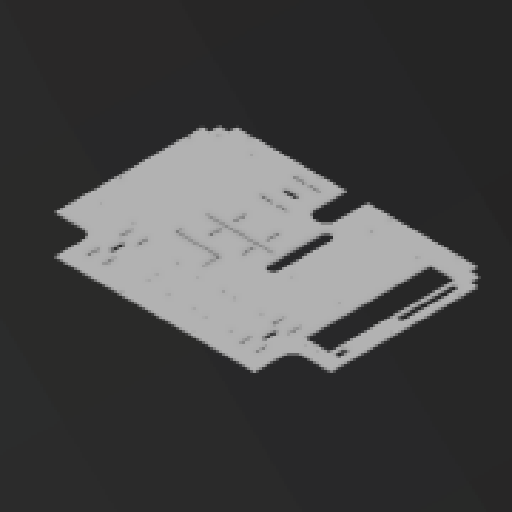
# Autodesk Inventor part: BasePlate
Saved by Autodesk Inventor 2023.2 (Build 272271000, 271)
## iProperties
Created: 2020-05-08
Part Number: BasePlate
Material: Aluminum 6061
Document SubType Name: Modeling
Designer: Remo
Mass: 4435.74 g
Surface Area: 3861.35 cm^2
Volume: 565.063 cm^3
Density: 2.7 g/cm^3
Appearance: Aluminum - Dark
Description: LaserTeileOnline / 3mm Aluminum / Base Plate
Author: Remo
Revision Number: 1
Autodesk Inventor part; units mm, degrees
ref_plane "YZ Plane" through (0, 0, 0) normal (1, 0, 0) x (0, 1, 0)
ref_plane "XZ Plane" through (0, 0, 0) normal (0, 1, 0) x (-1, 0, 0)
ref_plane "XY Plane" through (0, 0, 0) normal (0, 0, 1) x (1, 0, 0)
sketch "Sketch1" plane through (0, 0, 0) normal (0, 0, 1) x (1, 0, 0)
  line L0 (-412.8165, 301.8597) -> (87.1835, 301.8597) projected
  line L1 (-427.8165, 301.8597) -> (-412.8165, 301.8597) projected
  line L2 (-427.8165, 286.8597) -> (-427.8165, 301.8597) projected
  line L3 (-427.8165, -73.1403) -> (-427.8165, 286.8597) projected
  line L4 (-412.8165, 286.8597) -> (-427.8165, 286.8597) projected
  line L5 (-412.8165, 286.8597) -> (-427.8165, 286.8597) projected
  line L6 (-412.8165, 301.8597) -> (-412.8165, 286.8597) projected
  line L7 (-427.8165, 301.8597) -> (-412.8165, 301.8597) projected
  line L8 (-427.8165, 286.8597) -> (-427.8165, 301.8597) projected
  line L9 (-412.8165, -88.1403) -> (-412.8165, -73.1403) projected
  line L10 (-412.8165, -73.1403) -> (-427.8165, -73.1403) projected
  line L11 (-427.8165, -88.1403) -> (-427.8165, -73.1403) projected
  line L12 (-412.8165, -88.1403) -> (-427.8165, -88.1403) projected
  line L13 (-412.8165, -73.1403) -> (-412.8165, 286.8597) projected
  line L14 (87.1835, -73.1403) -> (-412.8165, -73.1403) projected
  line L15 (87.1835, -88.1403) -> (-412.8165, -88.1403) projected
  line L16 (102.1835, -88.1403) -> (102.1835, -73.1403) projected
  line L17 (102.1835, -73.1403) -> (87.1835, -73.1403) projected
  line L18 (87.1835, -88.1403) -> (87.1835, -73.1403) projected
  line L19 (102.1835, -88.1403) -> (87.1835, -88.1403) projected
  line L20 (87.1835, -73.1403) -> (87.1835, 286.8597) projected
  line L21 (102.1835, -73.1403) -> (102.1835, 286.8597) projected
  line L22 (87.1835, 286.8597) -> (102.1835, 286.8597) projected
  line L23 (102.1835, 286.8597) -> (102.1835, 301.8597) projected
  line L24 (87.1835, 301.8597) -> (102.1835, 301.8597) projected
  line L25 (87.1835, 286.8597) -> (87.1835, 301.8597) projected
  line L26 (87.1835, 286.8597) -> (-412.8165, 286.8597) projected
  line L27 (-312.8165, -73.1403) -> (-312.8165, 286.8597) projected
  line L28 (-297.8165, -73.1403) -> (-297.8165, 286.8597) projected
  line L29 (-12.8165, -73.1403) -> (-12.8165, 286.8597) projected
  line L30 (-27.8165, -73.1403) -> (-27.8165, 286.8597) projected
  line L31 (-425.8165, -71.1403) -> (-410.8165, -71.1403)
  line L32 (-410.8165, -71.1403) -> (-410.8165, -86.1403)
  line L33 (-410.8165, -86.1403) -> (85.1835, -86.1403)
  line L34 (85.1835, -86.1403) -> (85.1835, -71.1403)
  line L35 (85.1835, -71.1403) -> (100.1835, -71.1403)
  line L36 (100.1835, -71.1403) -> (100.1835, 284.8597)
  line L37 (100.1835, 284.8597) -> (85.1835, 284.8597)
  line L38 (85.1835, 284.8597) -> (85.1835, 299.8597)
  line L39 (85.1835, 299.8597) -> (-410.8165, 299.8597)
  line L40 (-410.8165, 299.8597) -> (-410.8165, 284.8597)
  line L41 (-410.8165, 284.8597) -> (-425.8165, 284.8597)
  line L42 (-425.8165, 284.8597) -> (-425.8165, -71.1403)
  point P0 (0, 0)
  dimension "d2" = 2
  dimension "d3" = 2
  dimension "d4" = 2
  dimension "d5" = 2
  dimension "d6" = 2
  dimension "d7" = 2
  dimension "d8" = 2
  dimension "d9" = 2
  dimension "d10" = 2
  dimension "d11" = 2
  dimension "d12" = 2
  dimension "d13" = 2
  constraints: 24 end point, 7 perpendicular, 4 parallel, 1 horizontal
  measures "d2" distance between parallel lines of L10 L31
  measures "d3" distance between parallel lines of L3 L42
  measures "d4" distance between parallel lines of L9 L32
  measures "d5" distance between parallel lines of L15 L33
  measures "d6" distance between parallel lines of L34 L18
  measures "d7" distance between parallel lines of L17 L35
  measures "d8" distance between parallel lines of L21 L36
  measures "d9" distance between parallel lines of L22 L37
  measures "d10" distance between parallel lines of L25 L38
  measures "d11" distance between parallel lines of L0 L39
  measures "d12" distance between parallel lines of L6 L40
  measures "d13" distance between parallel lines of L4 L41
extrude "Extrusion1" add sketch "Sketch1" along normal blind 3 contours L41 L40 L26 L27 L14 L32 L31 L13 | L13 L31 L42 L41 | L40 L39 L38 L26 | L37 L36 L35 L20 | L20 L35 L34 L14 L29 L26 L38 L37 | L26 L28 L14 L27 | L29 L14 L30 L26 | L26 L30 L14 L28 | L14 L34 L33 L32
sketch "Sketch3" plane through (0, 0, 3) normal (0, 0, 1) x (1, 0, 0)
  line L0 (100.1835, -71.1403) -> (100.1835, 284.8597) projected
  line L1 (-425.8165, 284.8597) -> (-425.8165, -71.1403) projected
  line L2 (-425.8165, -71.1403) -> (-410.8165, -71.1403) projected
  line L3 (-410.8165, 284.8597) -> (-425.8165, 284.8597) projected
  line L4 (85.1835, -86.1403) -> (85.1835, -71.1403) projected
  line L5 (-410.8165, 299.8597) -> (-410.8165, 284.8597) projected
  line L6 (-410.8165, -86.1403) -> (85.1835, -86.1403) projected
  line L7 (85.1835, 299.8597) -> (-410.8165, 299.8597) projected
  point P0 (0, 0)
  point P1 (94.6835, -21.1403)
  point P2 (94.6835, 106.8597)
  point P3 (94.6835, 234.8597)
  point P4 (-420.3165, 234.8597)
  point P5 (-420.3165, 106.8597)
  point P6 (-420.3165, -21.1403)
  point P7 (35.1835, -80.6403)
  point P8 (-94.8165, -80.6403)
  point P9 (-230.8165, -80.6403)
  point P10 (-360.8165, -80.6403)
  point P11 (-360.8165, 294.3597)
  point P12 (-230.8165, 294.3597)
  point P13 (-94.8165, 294.3597)
  point P14 (35.1835, 294.3597)
  dimension "d18" = 5.5
  dimension "d19" = 5.5
  dimension "d20" = 50
  dimension "d21" = 50
  dimension "d22" = 356
  dimension "d23" = 178
  dimension "d24" = 50
  dimension "d25" = 50
  dimension "d26" = 5.5
  dimension "d27" = 5.5
  dimension "d28" = 180
  dimension "d29" = 180
  constraints: 9 horizontal alignment, 8 vertical alignment
  measures "d18" distance from line of L0 point (94.684, -21.14)
  measures "d19" distance from line of L1 point (-420.316, -21.14)
  measures "d20" distance from line of L2 point (-420.316, -21.14)
  measures "d21" distance from line of L3 point (-420.316, 234.86)
  measures "d22" distance of L1.start L1.end
  measures "d23" distance from line of L2 point (-420.316, 106.86)
  measures "d24" distance from line of L4 point (35.184, -80.64)
  measures "d25" distance from line of L5 point (-360.816, 294.36)
  measures "d26" distance from line of L6 point (35.184, -80.64)
  measures "d27" distance from line of L7 point (35.184, 294.36)
  measures "d28" horizontal distance of L6.start point (-230.816, -80.64)
  measures "d29" distance from line of L4 point (-94.816, -80.64)
hole "FrameMountHoles" at (94.6835, -21.1403, 3) at (94.6835, 106.8597, 3) at (94.6835, 234.8597, 3) at (-420.3165, 234.8597, 3) at (-420.3165, 106.8597, 3) at (-420.3165, -21.1403, 3) at (35.1835, -80.6403, 3) at (-94.8165, -80.6403, 3) at (-230.8165, -80.6403, 3) at (-360.8165, -80.6403, 3) at (-360.8165, 294.3597, 3) at (-230.8165, 294.3597, 3) at (-94.8165, 294.3597, 3) at (35.1835, 294.3597, 3) direction (0, 0, -1) diameter 4 depth 8 tip angle 118
sketch "Sketch10" plane through (0, 0, 3) normal (0, 0, 1) x (1, 0, 0)
  circle A0 centre (-94.8165, 294.3597) radius 2 projected
  circle A1 centre (-360.8165, 294.3597) radius 2 projected
  circle A2 centre (-230.8165, -80.6403) radius 2 projected
  circle A3 centre (35.1835, -80.6403) radius 2 projected
  circle A4 centre (-420.3165, 106.8597) radius 2 projected
  circle A5 centre (94.6835, 234.8597) radius 2 projected
  circle A6 centre (94.6835, -21.1403) radius 2 projected
  circle A7 centre (94.6835, 106.8597) radius 2 projected
  circle A8 centre (-420.3165, 234.8597) radius 2 projected
  circle A9 centre (-420.3165, -21.1403) radius 2 projected
  circle A10 centre (-94.8165, -80.6403) radius 2 projected
  circle A11 centre (-360.8165, -80.6403) radius 2 projected
  circle A12 centre (-230.8165, 294.3597) radius 2 projected
  circle A13 centre (35.1835, 294.3597) radius 2 projected
  line L0 (-425.8165, -71.1403) -> (-410.8165, -71.1403) projected
  line L1 (-410.8165, -71.1403) -> (-410.8165, -86.1403) projected
  line L2 (-410.8165, -86.1403) -> (85.1835, -86.1403) projected
  line L3 (85.1835, -86.1403) -> (85.1835, -71.1403) projected
  line L4 (85.1835, -71.1403) -> (100.1835, -71.1403) projected
  line L5 (100.1835, -71.1403) -> (100.1835, 284.8597) projected
  line L6 (100.1835, 284.8597) -> (85.1835, 284.8597) projected
  line L7 (85.1835, 284.8597) -> (85.1835, 299.8597) projected
  line L8 (85.1835, 299.8597) -> (-410.8165, 299.8597) projected
  line L9 (-410.8165, 299.8597) -> (-410.8165, 284.8597) projected
  line L10 (-410.8165, 284.8597) -> (-425.8165, 284.8597) projected
  line L11 (-425.8165, 284.8597) -> (-425.8165, -71.1403) projected
  line L12 (100.1835, -71.1403) -> (100.1835, 284.8597) projected
  line L13 (85.1835, 284.8597) -> (100.1835, 284.8597)
  line L14 (100.1835, 284.8597) -> (100.1835, 266.8597)
  line L15 (100.1835, 266.8597) -> (85.1835, 266.8597)
  line L16 (85.1835, 266.8597) -> (85.1835, 284.8597)
  line L17 (85.1835, 284.8597) -> (67.1835, 284.8597)
  line L18 (67.1835, 284.8597) -> (67.1835, 299.8597)
  line L19 (67.1835, 299.8597) -> (85.1835, 299.8597)
  line L20 (85.1835, 299.8597) -> (85.1835, 284.8597)
  line L21 (-410.8165, 284.8597) -> (-392.8165, 284.8597)
  line L22 (-392.8165, 284.8597) -> (-392.8165, 299.8597)
  line L23 (-392.8165, 299.8597) -> (-410.8165, 299.8597)
  line L24 (-410.8165, 299.8597) -> (-410.8165, 284.8597)
  line L25 (-410.8165, 284.8597) -> (-425.8165, 284.8597)
  line L26 (-425.8165, 284.8597) -> (-425.8165, 266.8597)
  line L27 (-425.8165, 266.8597) -> (-410.8165, 266.8597)
  line L28 (-410.8165, 266.8597) -> (-410.8165, 284.8597)
  line L29 (-410.8165, -71.1403) -> (-425.8165, -71.1403)
  line L30 (-425.8165, -71.1403) -> (-425.8165, -53.1403)
  line L31 (-425.8165, -53.1403) -> (-410.8165, -53.1403)
  line L32 (-410.8165, -53.1403) -> (-410.8165, -71.1403)
  line L33 (-410.8165, -71.1403) -> (-392.8165, -71.1403)
  line L34 (-392.8165, -71.1403) -> (-392.8165, -86.1403)
  line L35 (-392.8165, -86.1403) -> (-410.8165, -86.1403)
  line L36 (-410.8165, -86.1403) -> (-410.8165, -71.1403)
  line L37 (-410.8165, -86.1403) -> (85.1835, -86.1403) projected
  line L38 (85.1835, -71.1403) -> (67.1835, -71.1403)
  line L39 (67.1835, -71.1403) -> (67.1835, -86.1403)
  line L40 (67.1835, -86.1403) -> (85.1835, -86.1403)
  line L41 (85.1835, -86.1403) -> (85.1835, -71.1403)
  line L42 (85.1835, -71.1403) -> (100.1835, -71.1403)
  line L43 (100.1835, -71.1403) -> (100.1835, -53.1403)
  line L44 (100.1835, -53.1403) -> (85.1835, -53.1403)
  line L45 (85.1835, -53.1403) -> (85.1835, -71.1403)
  point P0 (0, 0)
  dimension "d78" = 18
  constraints: 64 end point, 16 parallel, 8 horizontal, 8 perpendicular, 8 point on line, 7 equal length
  measures "d78" distance of L3.end L38.end
extrude "TriCuts" cut sketch "Sketch10" against normal through all contours L11 L31 L32 L0 | L33 L34 L2 L1 | L11 L10 L28 L27 | L39 L38 L3 L2 | L9 L8 L22 L21 | L45 L44 L5 L4 | L8 L7 L17 L18 | L15 L16 L6 L5
sketch "Sketch18" plane through (0, 0, 0) normal (0, 0, -1) x (-1, 0, 0)
  circle A0 centre (-35.1835, 294.3597) radius 2 projected
  circle A1 centre (230.8165, 294.3597) radius 2 projected
  circle A2 centre (360.8165, -80.6403) radius 2 projected
  circle A3 centre (94.8165, -80.6403) radius 2 projected
  circle A4 centre (420.3165, -21.1403) radius 2 projected
  circle A5 centre (420.3165, 234.8597) radius 2 projected
  circle A6 centre (-94.6835, 106.8597) radius 2 projected
  circle A7 centre (-94.6835, -21.1403) radius 2 projected
  circle A8 centre (-94.6835, 234.8597) radius 2 projected
  circle A9 centre (420.3165, 106.8597) radius 2 projected
  circle A10 centre (-35.1835, -80.6403) radius 2 projected
  circle A11 centre (230.8165, -80.6403) radius 2 projected
  circle A12 centre (360.8165, 294.3597) radius 2 projected
  circle A13 centre (94.8165, 294.3597) radius 2 projected
  line L0 (425.8165, 266.8597) -> (410.8165, 266.8597) projected
  line L1 (410.8165, 266.8597) -> (410.8165, 284.8597) projected
  line L2 (410.8165, 284.8597) -> (392.8165, 284.8597) projected
  line L3 (392.8165, 284.8597) -> (392.8165, 299.8597) projected
  line L4 (-67.1835, 299.8597) -> (392.8165, 299.8597) projected
  line L5 (-67.1835, 299.8597) -> (-67.1835, 284.8597) projected
  line L6 (-67.1835, 284.8597) -> (-85.1835, 284.8597) projected
  line L7 (-85.1835, 284.8597) -> (-85.1835, 266.8597) projected
  line L8 (-85.1835, 266.8597) -> (-100.1835, 266.8597) projected
  line L9 (-100.1835, -53.1403) -> (-100.1835, 266.8597) projected
  line L10 (-100.1835, -53.1403) -> (-85.1835, -53.1403) projected
  line L11 (-85.1835, -53.1403) -> (-85.1835, -71.1403) projected
  line L12 (-85.1835, -71.1403) -> (-67.1835, -71.1403) projected
  line L13 (-67.1835, -71.1403) -> (-67.1835, -86.1403) projected
  line L14 (392.8165, -86.1403) -> (-67.1835, -86.1403) projected
  line L15 (392.8165, -86.1403) -> (392.8165, -71.1403) projected
  line L16 (392.8165, -71.1403) -> (410.8165, -71.1403) projected
  line L17 (410.8165, -71.1403) -> (410.8165, -53.1403) projected
  line L18 (410.8165, -53.1403) -> (425.8165, -53.1403) projected
  line L19 (425.8165, 266.8597) -> (425.8165, -53.1403) projected
  circle A14 centre (-47.2571, -33.2139) radius 4 projected
  circle A15 centre (-47.2571, -33.2139) radius 20
  line L20 (-27.2571, -33.2139) -> (-27.2571, -86.1403)
  line L21 (392.8165, -86.1403) -> (-67.1835, -86.1403) projected
  line L22 (-47.2571, -13.2139) -> (-100.1835, -13.2139)
  line L23 (-100.1835, -53.1403) -> (-100.1835, 266.8597) projected
  circle A16 centre (372.89, -33.2139) radius 4 projected
  circle A17 centre (372.89, -33.2139) radius 20
  line L24 (372.89, -13.2139) -> (425.8165, -13.2139)
  line L25 (425.8165, 266.8597) -> (425.8165, -53.1403) projected
  line L26 (352.89, -33.2139) -> (352.89, -86.1403)
  line L27 (392.8165, -86.1403) -> (-67.1835, -86.1403) projected
  circle A18 centre (162.8165, 240.7787) radius 4 projected
  circle A19 centre (162.8165, 240.7787) radius 20
  line L28 (142.8165, 240.7787) -> (142.8165, 299.8597)
  line L29 (-67.1835, 299.8597) -> (392.8165, 299.8597) projected
  line L30 (182.8165, 240.7787) -> (182.8165, 299.8597)
  line L31 (-20.1835, 16.7861) -> (-67.1835, 16.7861)
  line L32 (-67.1835, 16.7861) -> (-67.1835, 256.7861)
  line L33 (-67.1835, 256.7861) -> (-20.1835, 256.7861)
  line L34 (-20.1835, 256.7861) -> (-20.1835, 16.7861)
  line L35 (-75.1835, 16.7861) -> (-85.1835, 16.7861)
  line L36 (-85.1835, 16.7861) -> (-85.1835, 36.7861)
  line L37 (-85.1835, 36.7861) -> (-75.1835, 36.7861)
  line L38 (-75.1835, 36.7861) -> (-75.1835, 16.7861)
  point P0 (0, 0)
  point P1 (352.89, -86.1403)
  dimension "d130" = 40
  dimension "d133" = 33
  dimension "d134" = 47
  dimension "d135" = 30
  dimension "d136" = 240
  dimension "d151" = 15
  dimension "d152" = 10
  dimension "d153" = 20
  constraints: 28 end point, 8 perpendicular, 6 point on circle, 6 point on line, 4 parallel, 4 tangent, 3 centre point, 3 coincident, 2 equal radius, 2 horizontal, 1 horizontal alignment
  measures "d130" diameter of A15
  measures "d133" distance between parallel lines of L23 L32
  measures "d134" distance of L31.start L31.end
  measures "d135" distance between parallel lines of L22 L31
  measures "d136" distance of L31.end L32.end
  measures "d151" distance between parallel lines of L23 L36
  measures "d152" distance of L35.start L35.end
  measures "d153" distance of L37.end L35.start
extrude "Cuts" cut sketch "Sketch18" against normal through all contours L19 L18 L17 L16 L15 L14 L26 A17 L24 | A17 | L30 A19 L28 L4 | L14 L13 L12 L11 L10 L9 L22 A15 L20 | A19 | A15 | A14 | A16 | A18 | L31 L32 L33 L34 | L35 L36 L37 L38
sketch "Sketch19" plane through (0, 0, 0) normal (0, 0, -1) x (-1, 0, 0)
  circle A0 centre (94.8165, 294.3597) radius 2 projected
  circle A1 centre (360.8165, 294.3597) radius 2 projected
  circle A2 centre (230.8165, -80.6403) radius 2 projected
  circle A3 centre (420.3165, 106.8597) radius 2 projected
  circle A4 centre (-94.6835, 234.8597) radius 2 projected
  circle A5 centre (-94.6835, 106.8597) radius 2 projected
  circle A6 centre (420.3165, 234.8597) radius 2 projected
  circle A7 centre (94.8165, -80.6403) radius 2 projected
  circle A8 centre (230.8165, 294.3597) radius 2 projected
  circle A9 centre (-35.1835, 294.3597) radius 2 projected
  line L0 (-67.1835, 16.7861) -> (-67.1835, 256.7861) projected
  line L1 (-67.1835, 256.7861) -> (-20.1835, 256.7861) projected
  line L2 (-20.1835, 256.7861) -> (-20.1835, 16.7861) projected
  line L3 (-20.1835, 16.7861) -> (-67.1835, 16.7861) projected
  line L4 (352.89, -86.1403) -> (352.89, -33.2139) projected
  arc A10 (372.89, -13.2139) -> (352.89, -33.2139) centre (372.89, -33.2139) ccw projected
  line L5 (372.89, -13.2139) -> (425.8165, -13.2139) projected
  line L6 (425.8165, 266.8597) -> (425.8165, -13.2139) projected
  line L7 (425.8165, 266.8597) -> (410.8165, 266.8597) projected
  line L8 (410.8165, 266.8597) -> (410.8165, 284.8597) projected
  line L9 (410.8165, 284.8597) -> (392.8165, 284.8597) projected
  line L10 (392.8165, 284.8597) -> (392.8165, 299.8597) projected
  line L11 (182.8165, 299.8597) -> (392.8165, 299.8597) projected
  line L12 (182.8165, 299.8597) -> (182.8165, 240.7787) projected
  arc A11 (142.8165, 240.7787) -> (182.8165, 240.7787) centre (162.8165, 240.7787) ccw projected
  line L13 (142.8165, 240.7787) -> (142.8165, 299.8597) projected
  line L14 (-67.1835, 299.8597) -> (142.8165, 299.8597) projected
  line L15 (-67.1835, 299.8597) -> (-67.1835, 284.8597) projected
  line L16 (-67.1835, 284.8597) -> (-85.1835, 284.8597) projected
  line L17 (-85.1835, 284.8597) -> (-85.1835, 266.8597) projected
  line L18 (-85.1835, 266.8597) -> (-100.1835, 266.8597) projected
  line L19 (-100.1835, -13.2139) -> (-100.1835, 266.8597) projected
  line L20 (-100.1835, -13.2139) -> (-47.2571, -13.2139) projected
  arc A12 (-27.2571, -33.2139) -> (-47.2571, -13.2139) centre (-47.2571, -33.2139) ccw projected
  line L21 (-27.2571, -33.2139) -> (-27.2571, -86.1403) projected
  line L22 (352.89, -86.1403) -> (-27.2571, -86.1403) projected
  line L23 (-20.1835, 16.7861) -> (-67.1835, 16.7861) projected
  point P0 (0, 0)
  point P1 (-32.6835, 4.7861)
  point P2 (-54.6835, 4.7861)
  point P3 (-43.6835, 12.7861)
  point P4 (-43.6835, 16.7861)
  point P5 (-43.6835, 16.7861)
  dimension "d137" = 12
  dimension "d138" = 4
  dimension "d139" = 22
  dimension "d140" = 11
  constraints: 2 midpoint, 1 horizontal alignment, 1 vertical alignment
  measures "d137" distance from line of L3 point (-32.684, 4.786)
  measures "d138" distance from line of L3 point (-43.684, 12.786)
  measures "d139" distance of point (-54.684, 4.786) point (-32.684, 4.786)
  measures "d140" horizontal distance of point (-43.684, 16.786) point (-54.684, 4.786)
hole "Drag Chain Z" at (32.6835, 4.7861, 0) at (54.6835, 4.7861, 0) at (43.6835, 12.7861, 0) direction (0, 0, 1) diameter 2.8 end through all
sketch "Sketch21" plane through (0, 0, 0) normal (0, 0, -1) x (-1, 0, 0)
  circle A0 centre (32.395, 19.3597) radius 1.75 projected
  circle A1 centre (2.395, 19.3597) radius 1.75 projected
  circle A2 centre (17.395, -12.1403) radius 2.5 projected
  circle A3 centre (32.395, -43.6403) radius 1.75 projected
  circle A4 centre (2.395, -43.6403) radius 1.75 projected
  circle A5 centre (323.2379, -43.6403) radius 1.75 projected
  circle A6 centre (293.2379, -43.6403) radius 1.75 projected
  circle A7 centre (308.2379, -12.1403) radius 2.5 projected
  circle A8 centre (293.2379, 19.3597) radius 1.75 projected
  circle A9 centre (323.2379, 19.3597) radius 1.75 projected
  circle A10 centre (245.8164, 272.3597) radius 1.75 projected
  circle A11 centre (215.8164, 272.3597) radius 1.75 projected
  circle A12 centre (230.8164, 240.8597) radius 2.5 projected
  circle A13 centre (245.8164, 209.3597) radius 1.75 projected
  circle A14 centre (215.8164, 209.3597) radius 1.75 projected
  line L0 (205.8164, 272.3597) -> (225.8164, 272.3597) construction
  line L1 (205.8164, 270.6097) -> (225.8164, 270.6097)
  line L2 (225.8164, 274.1097) -> (205.8164, 274.1097)
  arc A15 (205.8164, 274.1097) -> (205.8164, 270.6097) centre (205.8164, 272.3597) ccw
  arc A16 (225.8164, 270.6097) -> (225.8164, 274.1097) centre (225.8164, 272.3597) ccw
  line L3 (235.8164, 272.3597) -> (255.8164, 272.3597) construction
  line L4 (235.8164, 270.6097) -> (255.8164, 270.6097)
  line L5 (255.8164, 274.1097) -> (235.8164, 274.1097)
  arc A17 (235.8164, 274.1097) -> (235.8164, 270.6097) centre (235.8164, 272.3597) ccw
  arc A18 (255.8164, 270.6097) -> (255.8164, 274.1097) centre (255.8164, 272.3597) ccw
  line L6 (235.8164, 209.3597) -> (255.8164, 209.3597) construction
  line L7 (235.8164, 207.6097) -> (255.8164, 207.6097)
  line L8 (255.8164, 211.1097) -> (235.8164, 211.1097)
  arc A19 (235.8164, 211.1097) -> (235.8164, 207.6097) centre (235.8164, 209.3597) ccw
  arc A20 (255.8164, 207.6097) -> (255.8164, 211.1097) centre (255.8164, 209.3597) ccw
  line L9 (205.8164, 209.3597) -> (225.8164, 209.3597) construction
  line L10 (205.8164, 207.6097) -> (225.8164, 207.6097)
  line L11 (225.8164, 211.1097) -> (205.8164, 211.1097)
  arc A21 (205.8164, 211.1097) -> (205.8164, 207.6097) centre (205.8164, 209.3597) ccw
  arc A22 (225.8164, 207.6097) -> (225.8164, 211.1097) centre (225.8164, 209.3597) ccw
  line L12 (220.8164, 240.8597) -> (240.8164, 240.8597) construction
  line L13 (220.8164, 236.8597) -> (240.8164, 236.8597)
  line L14 (240.8164, 244.8597) -> (220.8164, 244.8597)
  arc A23 (220.8164, 244.8597) -> (220.8164, 236.8597) centre (220.8164, 240.8597) ccw
  arc A24 (240.8164, 236.8597) -> (240.8164, 244.8597) centre (240.8164, 240.8597) ccw
  line L15 (293.2379, 9.3597) -> (293.2379, 29.3597) construction
  line L16 (291.4879, 9.3597) -> (291.4879, 29.3597)
  line L17 (294.9879, 29.3597) -> (294.9879, 9.3597)
  arc A25 (291.4879, 9.3597) -> (294.9879, 9.3597) centre (293.2379, 9.3597) ccw
  arc A26 (294.9879, 29.3597) -> (291.4879, 29.3597) centre (293.2379, 29.3597) ccw
  line L18 (323.2379, 29.3597) -> (323.2379, 9.3597) construction
  line L19 (324.9879, 29.3597) -> (324.9879, 9.3597)
  line L20 (321.4879, 9.3597) -> (321.4879, 29.3597)
  arc A27 (324.9879, 29.3597) -> (321.4879, 29.3597) centre (323.2379, 29.3597) ccw
  arc A28 (321.4879, 9.3597) -> (324.9879, 9.3597) centre (323.2379, 9.3597) ccw
  line L21 (308.2379, -22.1403) -> (308.2379, -2.1403) construction
  line L22 (312.2379, -22.1403) -> (312.2379, -2.1403)
  line L23 (304.2379, -2.1403) -> (304.2379, -22.1403)
  arc A29 (304.2379, -22.1403) -> (312.2379, -22.1403) centre (308.2379, -22.1403) ccw
  arc A30 (312.2379, -2.1403) -> (304.2379, -2.1403) centre (308.2379, -2.1403) ccw
  line L24 (293.2379, -53.6403) -> (293.2379, -33.6403) construction
  line L25 (294.9879, -53.6403) -> (294.9879, -33.6403)
  line L26 (291.4879, -33.6403) -> (291.4879, -53.6403)
  arc A31 (291.4879, -53.6403) -> (294.9879, -53.6403) centre (293.2379, -53.6403) ccw
  arc A32 (294.9879, -33.6403) -> (291.4879, -33.6403) centre (293.2379, -33.6403) ccw
  line L27 (323.2379, -53.6403) -> (323.2379, -33.6403) construction
  line L28 (321.4879, -53.6403) -> (321.4879, -33.6403)
  line L29 (324.9879, -33.6403) -> (324.9879, -53.6403)
  arc A33 (321.4879, -53.6403) -> (324.9879, -53.6403) centre (323.2379, -53.6403) ccw
  arc A34 (324.9879, -33.6403) -> (321.4879, -33.6403) centre (323.2379, -33.6403) ccw
  line L30 (17.395, -22.1403) -> (17.395, -2.1403) construction
  line L31 (13.395, -22.1403) -> (13.395, -2.1403)
  line L32 (21.395, -2.1403) -> (21.395, -22.1403)
  arc A35 (13.395, -22.1403) -> (21.395, -22.1403) centre (17.395, -22.1403) ccw
  arc A36 (21.395, -2.1403) -> (13.395, -2.1403) centre (17.395, -2.1403) ccw
  line L33 (32.395, 9.3597) -> (32.395, 29.3597) construction
  line L34 (30.645, 9.3597) -> (30.645, 29.3597)
  line L35 (34.145, 29.3597) -> (34.145, 9.3597)
  arc A37 (30.645, 9.3597) -> (34.145, 9.3597) centre (32.395, 9.3597) ccw
  arc A38 (34.145, 29.3597) -> (30.645, 29.3597) centre (32.395, 29.3597) ccw
  line L36 (2.395, 9.3597) -> (2.395, 29.3597) construction
  line L37 (0.645, 9.3597) -> (0.645, 29.3597)
  line L38 (4.145, 29.3597) -> (4.145, 9.3597)
  arc A39 (0.645, 9.3597) -> (4.145, 9.3597) centre (2.395, 9.3597) ccw
  arc A40 (4.145, 29.3597) -> (0.645, 29.3597) centre (2.395, 29.3597) ccw
  line L39 (2.395, -53.6403) -> (2.395, -33.6403) construction
  line L40 (0.645, -53.6403) -> (0.645, -33.6403)
  line L41 (4.145, -33.6403) -> (4.145, -53.6403)
  arc A41 (0.645, -53.6403) -> (4.145, -53.6403) centre (2.395, -53.6403) ccw
  arc A42 (4.145, -33.6403) -> (0.645, -33.6403) centre (2.395, -33.6403) ccw
  line L42 (32.395, -53.6403) -> (32.395, -33.6403) construction
  line L43 (30.645, -53.6403) -> (30.645, -33.6403)
  line L44 (34.145, -33.6403) -> (34.145, -53.6403)
  arc A43 (30.645, -53.6403) -> (34.145, -53.6403) centre (32.395, -53.6403) ccw
  arc A44 (34.145, -33.6403) -> (30.645, -33.6403) centre (32.395, -33.6403) ccw
  point P0 (0, 0)
  dimension "d154" = 4
  dimension "d155" = 20
  constraints: 120 end point, 60 point on circle, 60 tangent, 30 centre point, 20 parallel, 15 midpoint, 14 equal length, 14 equal radius, 6 point on line, 2 horizontal, 2 vertical
  measures "d154" radius of A24
  measures "d155" distance of L1.start L1.end
extrude "Extrusion10" cut sketch "Sketch21" against normal through all contours A0 | L35 A37 L34 A0 | A0 L34 A38 L35 | A1 | L38 A39 L37 A1 | A1 L37 A40 L38 | A2 | A3 | L44 A43 L43 A3 | A3 L43 A44 L44 | A4 | L41 A41 L40 A4 | A4 L40 A42 L41 | A5 | L29 A33 L28 A5 | A5 L28 A34 L29 | A6 | L25 A31 L26 A6 | A6 L26 A32 L25 | A7 | A8 | L17 A25 L16 A8 | A8 L16 A26 L17 | A9 | L19 A28 L20 A9 | A9 L20 A27 L19 | A10 | A10 L5 A18 L4 | A10 L4 A17 L5 | A11 | A11 L2 A16 L1 | A11 L1 A15 L2 | A12 | A13 | A13 L8 A20 L7 | A13 L7 A19 L8 | A14 | A14 L11 A22 L10 | A14 L10 A21 L11 | A23 L14 A24 L13 | A29 L23 A30 L22 | L31 A36 L32 A35
sketch "Sketch22" plane through (0, 0, 0) normal (0, 0, -1) x (-1, 0, 0)
  circle A0 centre (66.3165, 12.3597) radius 1.25 projected
  circle A1 centre (115.3165, 12.3597) radius 1.25 projected
  circle A2 centre (115.3165, -45.6403) radius 1.25 projected
  circle A3 centre (66.3165, -45.6403) radius 1.25 projected
  circle A4 centre (137.3165, -45.6403) radius 1.25 projected
  circle A5 centre (186.3165, -45.6403) radius 1.25 projected
  circle A6 centre (186.3165, 12.3597) radius 1.25 projected
  circle A7 centre (137.3165, 12.3597) radius 1.25 projected
  circle A8 centre (244.3808, 150.2472) radius 2.2479 projected
  arc A9 (246.6287, 102.6222) -> (242.1329, 102.6222) centre (244.3808, 102.6222) ccw projected
  arc A10 (184.3123, 102.6222) -> (179.8165, 102.6222) centre (182.0644, 102.6222) ccw projected
  circle A11 centre (182.0644, 150.2472) radius 2.2479 projected
  circle A12 centre (97.7753, 252.8597) radius 3 projected
  circle A13 centre (7.7753, 252.8597) radius 3 projected
  circle A14 centre (7.7753, 102.8597) radius 3 projected
  circle A15 centre (97.7753, 102.8597) radius 3 projected
  arc A16 (399.8178, 266.8597) -> (403.8178, 266.8597) centre (401.8178, 266.8597) ccw projected
  arc A17 (336.8178, 266.8597) -> (340.8178, 266.8597) centre (338.8178, 266.8597) ccw projected
  arc A18 (340.8178, 40.8597) -> (336.8178, 40.8597) centre (338.8178, 40.8597) ccw projected
  arc A19 (403.8178, 40.8597) -> (399.8178, 40.8597) centre (401.8178, 40.8597) ccw projected
  circle A20 centre (230.4165, 16.3597) radius 1.5 projected
  circle A21 centre (230.4165, -38.6403) radius 1.5 projected
  circle A22 centre (230.4165, -22.7403) radius 2.2377
  line L0 (125.2753, 102.8597) -> (125.2753, 202.8597) construction
  line L1 (135.2753, 102.8597) -> (135.2753, 202.8597)
  line L2 (115.2753, 202.8597) -> (115.2753, 102.8597)
  arc A23 (115.2753, 102.8597) -> (135.2753, 102.8597) centre (125.2753, 102.8597) ccw
  arc A24 (135.2753, 202.8597) -> (115.2753, 202.8597) centre (125.2753, 202.8597) ccw
  line L3 (-79.6835, 241.7861) -> (-79.6835, 141.7861) construction
  line L4 (-74.1835, 241.7861) -> (-74.1835, 141.7861)
  line L5 (-85.1835, 141.7861) -> (-85.1835, 241.7861)
  arc A25 (-74.1835, 241.7861) -> (-85.1835, 241.7861) centre (-79.6835, 241.7861) ccw
  arc A26 (-85.1835, 141.7861) -> (-74.1835, 141.7861) centre (-79.6835, 141.7861) ccw
  line L6 (-67.1835, 16.7861) -> (-67.1835, 256.7861) projected
  line L7 (-100.1835, -13.2139) -> (-100.1835, 266.8597) projected
  point P0 (0, 0)
  point P1 (125.2753, 152.8597)
  point P2 (-79.6835, 191.7861)
  dimension "d158" = 39.1
  dimension "d161" = 100
  dimension "d162" = 27.5
  dimension "d163" = 10
  dimension "d164" = 7
  dimension "d165" = 15
  dimension "d166" = 15
  constraints: 16 end point, 8 point on circle, 8 tangent, 5 centre point, 3 parallel, 2 midpoint, 2 vertical, 1 horizontal alignment, 1 vertical alignment
  measures "d158" distance of A22.centre A20.centre
  measures "d161" distance of L0.start L0.end
  measures "d162" distance of A15.centre L0.start
  measures "d163" radius of A23
  measures "d164" distance between parallel lines of L4 L6
  measures "d165" distance between parallel lines of L7 L5
  measures "d166" vertical distance of L6.end L3.start
extrude "Extrusion11" cut sketch "Sketch22" against normal through all contours A23 L2 A24 L1 | L4 A26 L5 A25
sketch "Sketch25" plane through (0, 0, 0) normal (0, 0, -1) x (-1, 0, 0)
  line L0 (115.2753, 102.8597) -> (115.2753, 202.8597) projected
  arc A0 (135.2753, 202.8597) -> (115.2753, 202.8597) centre (125.2753, 202.8597) ccw projected
  line L1 (135.2753, 202.8597) -> (135.2753, 102.8597) projected
  arc A1 (115.2753, 102.8597) -> (135.2753, 102.8597) centre (125.2753, 102.8597) ccw projected
  arc A2 (-74.1835, 241.7861) -> (-85.1835, 241.7861) centre (-79.6835, 241.7861) ccw projected
  line L2 (-74.1835, 241.7861) -> (-74.1835, 141.7861) projected
  arc A3 (-85.1835, 141.7861) -> (-74.1835, 141.7861) centre (-79.6835, 141.7861) ccw projected
  line L3 (-85.1835, 141.7861) -> (-85.1835, 241.7861) projected
  arc A4 (30.645, 9.3597) -> (34.145, 9.3597) centre (32.395, 9.3597) ccw projected
  line L4 (30.645, 9.3597) -> (30.645, 29.3597) projected
  arc A5 (34.145, 29.3597) -> (30.645, 29.3597) centre (32.395, 29.3597) ccw projected
  line L5 (34.145, 29.3597) -> (34.145, 9.3597) projected
  arc A6 (291.4879, -53.6403) -> (294.9879, -53.6403) centre (293.2379, -53.6403) ccw projected
  line L6 (291.4879, -53.6403) -> (291.4879, -33.6403) projected
  arc A7 (294.9879, -33.6403) -> (291.4879, -33.6403) centre (293.2379, -33.6403) ccw projected
  line L7 (294.9879, -33.6403) -> (294.9879, -53.6403) projected
  arc A8 (235.8164, 211.1097) -> (235.8164, 207.6097) centre (235.8164, 209.3597) ccw projected
  line L8 (235.8164, 211.1097) -> (255.8164, 211.1097) projected
  arc A9 (255.8164, 207.6097) -> (255.8164, 211.1097) centre (255.8164, 209.3597) ccw projected
  line L9 (255.8164, 207.6097) -> (235.8164, 207.6097) projected
  line L10 (235.8164, 274.1097) -> (255.8164, 274.1097) projected
  arc A10 (255.8164, 270.6097) -> (255.8164, 274.1097) centre (255.8164, 272.3597) ccw projected
  line L11 (255.8164, 270.6097) -> (235.8164, 270.6097) projected
  arc A11 (235.8164, 274.1097) -> (235.8164, 270.6097) centre (235.8164, 272.3597) ccw projected
  arc A12 (205.8164, 211.1097) -> (205.8164, 207.6097) centre (205.8164, 209.3597) ccw projected
  line L12 (205.8164, 211.1097) -> (225.8164, 211.1097) projected
  arc A13 (225.8164, 207.6097) -> (225.8164, 211.1097) centre (225.8164, 209.3597) ccw projected
  line L13 (225.8164, 207.6097) -> (205.8164, 207.6097) projected
  line L14 (304.2379, -22.1403) -> (304.2379, -2.1403) projected
  arc A14 (312.2379, -2.1403) -> (304.2379, -2.1403) centre (308.2379, -2.1403) ccw projected
  line L15 (312.2379, -2.1403) -> (312.2379, -22.1403) projected
  arc A15 (304.2379, -22.1403) -> (312.2379, -22.1403) centre (308.2379, -22.1403) ccw projected
  line L16 (30.645, -53.6403) -> (30.645, -33.6403) projected
  arc A16 (34.145, -33.6403) -> (30.645, -33.6403) centre (32.395, -33.6403) ccw projected
  line L17 (34.145, -33.6403) -> (34.145, -53.6403) projected
  arc A17 (30.645, -53.6403) -> (34.145, -53.6403) centre (32.395, -53.6403) ccw projected
  arc A18 (4.145, 29.3597) -> (0.645, 29.3597) centre (2.395, 29.3597) ccw projected
  line L18 (4.145, 29.3597) -> (4.145, 9.3597) projected
  arc A19 (0.645, 9.3597) -> (4.145, 9.3597) centre (2.395, 9.3597) ccw projected
  line L19 (0.645, 9.3597) -> (0.645, 29.3597) projected
  line L20 (321.4879, -53.6403) -> (321.4879, -33.6403) projected
  arc A20 (324.9879, -33.6403) -> (321.4879, -33.6403) centre (323.2379, -33.6403) ccw projected
  line L21 (324.9879, -33.6403) -> (324.9879, -53.6403) projected
  arc A21 (321.4879, -53.6403) -> (324.9879, -53.6403) centre (323.2379, -53.6403) ccw projected
  arc A22 (324.9879, 29.3597) -> (321.4879, 29.3597) centre (323.2379, 29.3597) ccw projected
  line L22 (324.9879, 29.3597) -> (324.9879, 9.3597) projected
  arc A23 (321.4879, 9.3597) -> (324.9879, 9.3597) centre (323.2379, 9.3597) ccw projected
  line L23 (321.4879, 9.3597) -> (321.4879, 29.3597) projected
  arc A24 (205.8164, 274.1097) -> (205.8164, 270.6097) centre (205.8164, 272.3597) ccw projected
  line L24 (205.8164, 274.1097) -> (225.8164, 274.1097) projected
  arc A25 (225.8164, 270.6097) -> (225.8164, 274.1097) centre (225.8164, 272.3597) ccw projected
  line L25 (225.8164, 270.6097) -> (205.8164, 270.6097) projected
  line L26 (220.8164, 244.8597) -> (240.8164, 244.8597) projected
  arc A26 (240.8164, 236.8597) -> (240.8164, 244.8597) centre (240.8164, 240.8597) ccw projected
  line L27 (240.8164, 236.8597) -> (220.8164, 236.8597) projected
  arc A27 (220.8164, 244.8597) -> (220.8164, 236.8597) centre (220.8164, 240.8597) ccw projected
  line L28 (291.4879, 9.3597) -> (291.4879, 29.3597) projected
  arc A28 (294.9879, 29.3597) -> (291.4879, 29.3597) centre (293.2379, 29.3597) ccw projected
  line L29 (294.9879, 29.3597) -> (294.9879, 9.3597) projected
  arc A29 (291.4879, 9.3597) -> (294.9879, 9.3597) centre (293.2379, 9.3597) ccw projected
  arc A30 (0.645, -53.6403) -> (4.145, -53.6403) centre (2.395, -53.6403) ccw projected
  line L30 (0.645, -53.6403) -> (0.645, -33.6403) projected
  arc A31 (4.145, -33.6403) -> (0.645, -33.6403) centre (2.395, -33.6403) ccw projected
  line L31 (4.145, -33.6403) -> (4.145, -53.6403) projected
  arc A32 (13.395, -22.1403) -> (21.395, -22.1403) centre (17.395, -22.1403) ccw projected
  line L32 (13.395, -22.1403) -> (13.395, -2.1403) projected
  arc A33 (21.395, -2.1403) -> (13.395, -2.1403) centre (17.395, -2.1403) ccw projected
  line L33 (21.395, -2.1403) -> (21.395, -22.1403) projected
  circle A34 centre (-54.6835, 4.7861) radius 1.4 projected
  circle A35 centre (-32.6835, 4.7861) radius 1.4 projected
  circle A36 centre (-43.6835, 12.7861) radius 1.4 projected
  line L34 (142.8165, 240.7787) -> (142.8165, 299.8597) projected
  line L35 (-67.1835, 299.8597) -> (142.8165, 299.8597) projected
  line L36 (-67.1835, 299.8597) -> (-67.1835, 284.8597) projected
  line L37 (-67.1835, 284.8597) -> (-85.1835, 284.8597) projected
  line L38 (-85.1835, 284.8597) -> (-85.1835, 266.8597) projected
  line L39 (-85.1835, 266.8597) -> (-100.1835, 266.8597) projected
  line L40 (-100.1835, -13.2139) -> (-100.1835, 266.8597) projected
  line L41 (-100.1835, -13.2139) -> (-47.2571, -13.2139) projected
  arc A37 (-27.2571, -33.2139) -> (-47.2571, -13.2139) centre (-47.2571, -33.2139) ccw projected
  line L42 (-27.2571, -33.2139) -> (-27.2571, -86.1403) projected
  line L43 (352.89, -86.1403) -> (-27.2571, -86.1403) projected
  line L44 (352.89, -86.1403) -> (352.89, -33.2139) projected
  arc A38 (372.89, -13.2139) -> (352.89, -33.2139) centre (372.89, -33.2139) ccw projected
  line L45 (372.89, -13.2139) -> (425.8165, -13.2139) projected
  line L46 (425.8165, 266.8597) -> (425.8165, -13.2139) projected
  line L47 (425.8165, 266.8597) -> (410.8165, 266.8597) projected
  line L48 (410.8165, 266.8597) -> (410.8165, 284.8597) projected
  line L49 (410.8165, 284.8597) -> (392.8165, 284.8597) projected
  line L50 (392.8165, 284.8597) -> (392.8165, 299.8597) projected
  line L51 (182.8165, 299.8597) -> (392.8165, 299.8597) projected
  line L52 (182.8165, 299.8597) -> (182.8165, 240.7787) projected
  arc A39 (142.8165, 240.7787) -> (182.8165, 240.7787) centre (162.8165, 240.7787) ccw projected
  line L53 (-67.1835, 16.7861) -> (-67.1835, 256.7861) projected
  line L54 (-67.1835, 256.7861) -> (-20.1835, 256.7861) projected
  line L55 (-20.1835, 256.7861) -> (-20.1835, 16.7861) projected
  line L56 (-20.1835, 16.7861) -> (-67.1835, 16.7861) projected
  line L57 (-85.1835, 16.7861) -> (-85.1835, 36.7861) projected
  line L58 (-85.1835, 36.7861) -> (-75.1835, 36.7861) projected
  line L59 (-75.1835, 36.7861) -> (-75.1835, 16.7861) projected
  line L60 (-75.1835, 16.7861) -> (-85.1835, 16.7861) projected
  circle A40 centre (-35.1835, 294.3597) radius 2 projected
  circle A41 centre (230.8165, 294.3597) radius 2 projected
  circle A42 centre (94.8165, -80.6403) radius 2 projected
  circle A43 centre (420.3165, 234.8597) radius 2 projected
  circle A44 centre (-94.6835, 106.8597) radius 2 projected
  circle A45 centre (-94.6835, 234.8597) radius 2 projected
  circle A46 centre (420.3165, 106.8597) radius 2 projected
  circle A47 centre (230.8165, -80.6403) radius 2 projected
  circle A48 centre (360.8165, 294.3597) radius 2 projected
  circle A49 centre (94.8165, 294.3597) radius 2 projected
  line L61 (195.2379, 39.3597) -> (195.2379, 69.3597) construction
  line L62 (193.7379, 39.3597) -> (193.7379, 69.3597)
  line L63 (196.7379, 69.3597) -> (196.7379, 39.3597)
  arc A50 (193.7379, 39.3597) -> (196.7379, 39.3597) centre (195.2379, 39.3597) ccw
  arc A51 (196.7379, 69.3597) -> (193.7379, 69.3597) centre (195.2379, 69.3597) ccw
  line L64 (276.6058, 69.3597) -> (195.2379, 69.3597) construction
  line L65 (276.6058, 70.8597) -> (195.2379, 70.8597)
  line L66 (195.2379, 67.8597) -> (276.6058, 67.8597)
  arc A52 (276.6058, 67.8597) -> (276.6058, 70.8597) centre (276.6058, 69.3597) ccw
  arc A53 (195.2379, 70.8597) -> (195.2379, 67.8597) centre (195.2379, 69.3597) ccw
  line L67 (149.8394, 126.4347) -> (276.6058, 126.4347) construction
  line L68 (149.8394, 124.9347) -> (276.6058, 124.9347)
  line L69 (276.6058, 127.9347) -> (149.8394, 127.9347)
  arc A54 (149.8394, 127.9347) -> (149.8394, 124.9347) centre (149.8394, 126.4347) ccw
  arc A55 (276.6058, 124.9347) -> (276.6058, 127.9347) centre (276.6058, 126.4347) ccw
  line L70 (159.8394, 154.5018) -> (159.8394, 98.3676) projected
  line L71 (266.6058, 98.3676) -> (266.6058, 154.5018) projected
  line L72 (276.6058, 79.3597) -> (276.6058, 69.3597) construction
  line L73 (275.1058, 79.3597) -> (275.1058, 69.3597)
  line L74 (278.1058, 69.3597) -> (278.1058, 79.3597)
  arc A56 (278.1058, 79.3597) -> (275.1058, 79.3597) centre (276.6058, 79.3597) ccw
  arc A57 (275.1058, 69.3597) -> (278.1058, 69.3597) centre (276.6058, 69.3597) ccw
  point P0 (0, 0)
  point P1 (195.2379, 54.3597)
  point P2 (235.9218, 69.3597)
  point P3 (196.7379, 67.8597)
  point P4 (213.2226, 126.4347)
  point P5 (159.8394, 126.4347)
  point P6 (276.6058, 74.3597)
  point P7 (275.1058, 70.8597)
  dimension "d180" = 30
  dimension "d181" = 40
  dimension "d182" = 98
  dimension "d183" = 3
  dimension "d187" = 10
  dimension "d188" = 10
  dimension "d189" = 10
  constraints: 32 end point, 16 point on circle, 16 tangent, 8 centre point, 5 midpoint, 4 parallel, 3 equal radius, 2 vertical, 1 horizontal, 1 horizontal alignment, 1 perpendicular, 1 vertical alignment
  measures "d180" distance of L61.start L61.end
  measures "d181" distance from line of A28.centre L64
  measures "d182" distance from line of A28.centre L61
  measures "d183" distance between parallel lines of L62 L63
  measures "d187" distance from line of L70 L67.start
  measures "d188" distance from line of L71 L67.end
  measures "d189" distance of L72.start L64.start
extrude "Extrusion14" cut sketch "Sketch25" against normal through all contours L62 A53 L66 L63 A50 | A51 L63 L66 A53 | L65 L73 A57 L66 L63 A51 | L73 A56 L74 A52 L65 | L65 A52 A57 L73 | A54 L69 L70 L68 | L70 L69 L71 L68 | L71 L69 A55 L68
sketch "Sketch26" plane through (0, 0, 0) normal (0, 0, -1) x (-1, 0, 0)
  circle A0 centre (92.7753, 105.8597) radius 3 projected
  circle A1 centre (2.7753, 105.8597) radius 3 projected
  circle A2 centre (2.7753, 255.8597) radius 3 projected
  circle A3 centre (92.7753, 255.8597) radius 3 projected
  arc A4 (331.8178, 269.8597) -> (335.8178, 269.8597) centre (333.8178, 269.8597) ccw projected
  arc A5 (394.8178, 269.8597) -> (398.8178, 269.8597) centre (396.8178, 269.8597) ccw projected
  arc A6 (398.8178, 43.8597) -> (394.8178, 43.8597) centre (396.8178, 43.8597) ccw projected
  arc A7 (335.8178, 43.8597) -> (331.8178, 43.8597) centre (333.8178, 43.8597) ccw projected
  circle A8 centre (225.4165, 19.3597) radius 1.5 projected
  circle A9 centre (225.4165, -35.6403) radius 1.5 projected
  circle A10 centre (61.3165, 15.3597) radius 1.5 projected
  circle A11 centre (110.3165, 15.3597) radius 1.25 projected
  circle A12 centre (110.3165, -42.6403) radius 1.25 projected
  circle A13 centre (61.3165, -42.6403) radius 1.5 projected
  circle A14 centre (132.3165, -42.6403) radius 1.5 projected
  circle A15 centre (181.3165, -42.6403) radius 1.5 projected
  circle A16 centre (181.3165, 15.3597) radius 1.5 projected
  circle A17 centre (132.3165, 15.3597) radius 1.5 projected
  point P0 (0, 0)
  point P1 (225.4165, -19.7403)
  dimension "d190" = 39.1
  constraints: 1 vertical alignment
  measures "d190" distance of point (225.416, -19.74) A8.centre
hole "Hole9" at (-225.4165, -19.7403, 0) at (-2.7753, 255.8597, 0) at (-2.7753, 105.8597, 0) at (-92.7753, 105.8597, 0) at (-333.8178, 43.8597, 0) at (-396.8178, 43.8597, 0) at (-333.8178, 269.8597, 0) at (-396.8178, 269.8597, 0) at (-225.4165, -35.6403, 0) at (-225.4165, 19.3597, 0) at (-181.3165, 15.3597, 0) at (-132.3165, 15.3597, 0) at (-132.3165, -42.6403, 0) at (-181.3165, -42.6403, 0) at (-61.3165, -42.6403, 0) at (-61.3165, 15.3597, 0) at (-110.3165, 15.3597, 0) at (-110.3165, -42.6403, 0) at (-92.7753, 255.8597, 0) direction (0, 0, 1) diameter 3.5 depth 8 tip angle 118
sketch "Sketch27" plane through (0, 0, 0) normal (0, 0, -1) x (-1, 0, 0)
  circle A0 centre (177.0644, 153.2472) radius 2.2479 projected
  circle A1 centre (239.3808, 153.2472) radius 2.2479 projected
  arc A2 (241.6287, 105.6222) -> (237.1329, 105.6222) centre (239.3808, 105.6222) ccw projected
  arc A3 (179.3123, 105.6222) -> (174.8165, 105.6222) centre (177.0644, 105.6222) ccw projected
  line L0 (177.0644, 115.6222) -> (177.0644, 95.6222) construction
  line L1 (178.8144, 115.6222) -> (178.8144, 95.6222)
  line L2 (175.3144, 95.6222) -> (175.3144, 115.6222)
  arc A4 (178.8144, 115.6222) -> (175.3144, 115.6222) centre (177.0644, 115.6222) ccw
  arc A5 (175.3144, 95.6222) -> (178.8144, 95.6222) centre (177.0644, 95.6222) ccw
  line L3 (239.3808, 115.6222) -> (239.3808, 95.6222) construction
  line L4 (237.6308, 115.6222) -> (237.6308, 95.6222)
  line L5 (241.1308, 95.6222) -> (241.1308, 115.6222)
  arc A6 (241.1308, 115.6222) -> (237.6308, 115.6222) centre (239.3808, 115.6222) ccw
  arc A7 (237.6308, 95.6222) -> (241.1308, 95.6222) centre (239.3808, 95.6222) ccw
  line L6 (239.3808, 163.2472) -> (239.3808, 143.2472) construction
  line L7 (237.6308, 163.2472) -> (237.6308, 143.2472)
  line L8 (241.1308, 143.2472) -> (241.1308, 163.2472)
  arc A8 (241.1308, 163.2472) -> (237.6308, 163.2472) centre (239.3808, 163.2472) ccw
  arc A9 (237.6308, 143.2472) -> (241.1308, 143.2472) centre (239.3808, 143.2472) ccw
  line L9 (177.0644, 163.2472) -> (177.0644, 143.2472) construction
  line L10 (175.3144, 163.2472) -> (175.3144, 143.2472)
  line L11 (178.8144, 143.2472) -> (178.8144, 163.2472)
  arc A10 (178.8144, 163.2472) -> (175.3144, 163.2472) centre (177.0644, 163.2472) ccw
  arc A11 (175.3144, 143.2472) -> (178.8144, 143.2472) centre (177.0644, 143.2472) ccw
  point P0 (0, 0)
  dimension "d198" = 1.75
  dimension "d199" = 20
  constraints: 32 end point, 16 point on circle, 16 tangent, 8 centre point, 5 parallel, 4 midpoint, 3 equal length, 3 equal radius, 3 vertical
  measures "d198" radius of A5
  measures "d199" distance of L2.start L2.end
extrude "Extrusion15" cut sketch "Sketch27" against normal through all contours L11 A0 L10 | A0 L10 A10 L11 | L11 A11 L10 A0 | L8 A1 L7 | A1 L7 A8 L8 | L8 A9 L7 A1 | L5 A7 L4 A2 | A2 L4 A6 L5 | L1 A5 L2 A3 | A3 L2 A4 L1
equation "\"d4\" = d2"
equation "\"d5\" = d3"
equation "\"d6\" = d2"
equation "\"d7\" = d2"
equation "\"d8\" = d3"
equation "\"d9\" = d2"
equation "\"d10\" = d2"
equation "\"d11\" = d3"
equation "\"d12\" = d2"
equation "\"d13\" = d2"
equation "\"d19\" = d18"
equation "\"d23\" = 0.5 * d22"
equation "\"d26\" = d18"
equation "\"d27\" = d18"
equation "\"d29\" = d28"
body "Solid1"
